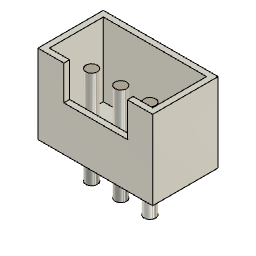
MLA30 v1.1 (Autodesk Fusion 360 archive; units mm, degrees)
design "JST-XH-3P"
Autodesk Fusion 360 part; units mm, degrees
note: some values were not read from the file. Set by a fixed rule: which face or edge a step refers to.
sketch "Esquisse1" plane through (0, 0, 0) normal (0, 0, 1) x (1, 0, 0) in component "JST-XH-3P"
  line L0 (6.25, 2.85) -> (-3.75, 2.85)
  line L1 (-3.75, 2.85) -> (-3.75, -2.85)
  line L2 (-3.75, -2.85) -> (6.25, -2.85)
  line L3 (6.25, -2.85) -> (6.25, 2.85)
  line L4 (6.25, 2.85) -> (-3.75, -2.85) construction
  line L5 (-3.75, 2.85) -> (6.25, -2.85) construction
  circle A0 centre (-1.27, -0.65) radius 0.5
  circle A1 centre (1.27, -0.65) radius 0.5
  circle A2 centre (3.81, -0.65) radius 0.5
  point P0 (1.25, 0)
  dimension "d6" = 10
  dimension "d7" = 5.7
  dimension "d8" = 1
  dimension "d11" = 5.08
  dimension "d12" = 0
  dimension "d13" = 2.48
  dimension "d20" = 2.2
  constraint horizontal L0
  constraint perpendicular L0 L1
  constraint parallel L0 L2
  constraint parallel L1 L3
  constraint coincident L4 P0
  constraint coincident L5 P0
  measures "d6" distance of L1.end L2.end
  measures "d7" distance of L0.end L1.end
  measures "d8" diameter of A0
  measures "d13" distance of L1 A0.centre
  measures "d20" distance of L2 A0.centre
extrude "Extrusion1" add sketch "Esquisse1" along normal blind 6.9 contours L0 L1 L2 L3 | A0 | A1 | A2 makes body 1 in component "JST-XH-3P"
shell "Coque1" thickness 0.5 removed faces 1 at (-0.4167, 0.95, 6.9) on bodies 1 in component "JST-XH-3P"
extrude "Extrusion2" add sketch "Esquisse1" against normal blind 3 separate body contours A0 | A1 | A2 makes body 2 at (-0.7706, -0.6749, -2) makes body 3 at (1.7694, -0.6749, -2) makes body 4 at (4.3094, -0.6749, -2) in component "JST-XH-3P"
sketch "Esquisse2" plane through (0, -2.85, 0) normal (0, -1, 0) x (1, 0, 0) in component "JST-XH-3P"
  line L0 (-3.75, 0) -> (6.25, 0)
  line L1 (6.25, 0) -> (6.25, 6.9)
  line L2 (6.25, 6.9) -> (-3.75, 6.9)
  line L3 (-3.75, 6.9) -> (-3.75, 0)
  line L4 (-1.4912, 6.9) -> (4.0488, 6.9)
  line L5 (4.0488, 6.9) -> (4.0488, 3.9)
  line L6 (4.0488, 3.9) -> (-1.4912, 3.9)
  line L7 (-1.4912, 3.9) -> (-1.4912, 6.9)
  dimension "d21" = 5.54
  dimension "d22" = 3
  constraint horizontal L4
  constraint vertical L5
  constraint horizontal L6
  constraint vertical L7
  constraint coincident L2 L4.start
  measures "d21" distance of L4.start L4.end
  measures "d22" distance of L4.start L6.end
extrude "Extrusion3" cut sketch "Esquisse2" against normal up to surface (0.5 mm away) contours L2 L4 L5 L6 L7 bodies 1 in component "JST-XH-3P"
extrude "Extrusion4" add sketch "Esquisse1" along normal blind 5.5 separate body contours A0 | A1 | A2 makes body 5 at (-0.7706, -0.6749, 3.6667) makes body 6 at (1.7694, -0.6749, 3.6667) makes body 7 at (4.3094, -0.6749, 3.6667) in component "JST-XH-3P"
component "JST-XH-3P" placed x (1, 0, 0) y (0, 1, 0) z (0, 0, 1) at (0, 0, 0)

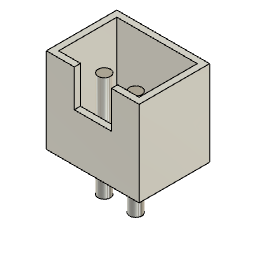
design "JST-XH-2P"
Autodesk Fusion 360 part; units mm, degrees
sketch "Esquisse1" plane through (0, 0, 0) normal (0, 0, 1) x (1, 0, 0) in component "JST-XH-2P"
  line L0 (3.75, 2.85) -> (-3.75, 2.85)
  line L1 (-3.75, 2.85) -> (-3.75, -2.85)
  line L2 (-3.75, -2.85) -> (3.75, -2.85)
  line L3 (3.75, -2.85) -> (3.75, 2.85)
  line L4 (3.75, 2.85) -> (-3.75, -2.85) construction
  line L5 (-3.75, 2.85) -> (3.75, -2.85) construction
  circle A0 centre (-1.27, -0.65) radius 0.5
  circle A1 centre (1.27, -0.65) radius 0.5
  dimension "d6" = 7.5
  dimension "d7" = 5.7
  dimension "d8" = 1
  dimension "d11" = 2.54
  dimension "d12" = 0
  dimension "d13" = 2.48
  dimension "d20" = 2.2
  constraint horizontal L0
  constraint perpendicular L0 L1
  constraint parallel L0 L2
  constraint parallel L1 L3
  constraint coincident L4 origin
  constraint coincident L5 origin
  measures "d6" distance of L1.end L2.end
  measures "d7" distance of L0.end L1.end
  measures "d8" diameter of A0
  measures "d13" distance of L1 A0.centre
  measures "d20" distance of L2 A0.centre
extrude "Extrusion1" add sketch "Esquisse1" along normal blind 6.9 contours L0 L1 L2 L3 | A0 | A1 makes body 1 in component "JST-XH-2P"
shell "Coque1" thickness 0.5 removed faces 1 at (-1.25, 0.95, 6.9) on bodies 1 in component "JST-XH-2P"
extrude "Extrusion2" add sketch "Esquisse1" against normal blind 3 separate body contours A0 | A1 makes body 2 at (-0.7706, -0.6749, -2) makes body 3 at (1.7694, -0.6749, -2) in component "JST-XH-2P"
sketch "Esquisse2" plane through (0, -2.85, 0) normal (0, -1, 0) x (1, 0, 0) in component "JST-XH-2P"
  line L0 (-3.75, 0) -> (3.75, 0)
  line L1 (3.75, 0) -> (3.75, 6.9)
  line L2 (3.75, 6.9) -> (-3.75, 6.9)
  line L3 (-3.75, 6.9) -> (-3.75, 0)
  line L4 (-1.4912, 6.9) -> (1.5088, 6.9)
  line L5 (1.5088, 6.9) -> (1.5088, 3.9)
  line L6 (1.5088, 3.9) -> (-1.4912, 3.9)
  line L7 (-1.4912, 3.9) -> (-1.4912, 6.9)
  dimension "d21" = 3
  dimension "d22" = 3
  constraint horizontal L4
  constraint vertical L5
  constraint horizontal L6
  constraint vertical L7
  constraint coincident L2 L4.start
  measures "d21" distance of L4.start L4.end
  measures "d22" distance of L4.start L6.end
extrude "Extrusion3" cut sketch "Esquisse2" against normal up to surface (0.5 mm away) contours L2 L4 L5 L6 L7 bodies 1 in component "JST-XH-2P"
extrude "Extrusion4" add sketch "Esquisse1" along normal blind 5.5 separate body contours A0 | A1 makes body 4 at (-0.7706, -0.6749, 3.6667) makes body 5 at (1.7694, -0.6749, 3.6667) in component "JST-XH-2P"
component "JST-XH-2P" placed x (1, 0, 0) y (0, 1, 0) z (0, 0, 1) at (0, 0, 0)

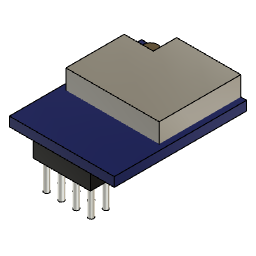
design "RA-02"
Autodesk Fusion 360 part; units mm, degrees
sketch "Esquisse1" plane through (0, 0, 0) normal (0, 0, 1) x (1, 0, 0) in component "LoRa RA-02"
  line L0 (0, 0) -> (18, 0)
  line L1 (18, 0) -> (18, -22.7)
  line L2 (18, -22.7) -> (0, -22.7)
  line L3 (0, -22.7) -> (0, 0)
  line L4 (1, 0) -> (17, 0)
  line L5 (17, 0) -> (17, -14)
  line L6 (17, -14) -> (1, -14)
  line L7 (1, -14) -> (1, 0)
  line L8 (13.9, -22.7) -> (4.1, -22.7)
  line L9 (4.1, -22.7) -> (4.1, -17.7)
  line L10 (4.1, -17.7) -> (13.9, -17.7)
  line L11 (13.9, -17.7) -> (13.9, -22.7)
  line L12 (1, 0) -> (6, 0)
  line L13 (6, 0) -> (6, -4)
  line L14 (6, -4) -> (1, -4)
  line L15 (1, -4) -> (1, 0)
  circle A0 centre (3.5142, -2) radius 1.25
  circle A1 centre (5.2, -21.5) radius 0.445
  circle A2 centre (7.74, -21.5) radius 0.445
  circle A3 centre (10.28, -21.5) radius 0.445
  circle A4 centre (12.82, -21.5) radius 0.445
  circle A5 centre (5.2, -18.96) radius 0.445
  circle A6 centre (7.74, -18.96) radius 0.445
  circle A7 centre (10.28, -18.96) radius 0.445
  circle A8 centre (12.82, -18.96) radius 0.445
  dimension "d1" = 18
  dimension "d2" = 22.7
  dimension "d3" = 16
  dimension "d4" = 14
  dimension "d5" = 9.8
  dimension "d6" = 5
  dimension "d7" = 5
  dimension "d8" = 4
  dimension "d9" = 2.5
  dimension "d18" = 0.89
  dimension "d21" = 7.62
  dimension "d22" = 2.54
  dimension "d23" = 1.2
  dimension "d24" = 1.1
  constraint horizontal L0
  constraint vertical L1
  constraint horizontal L2
  constraint vertical L3
  constraint coincident L0.start L3.end
  constraint horizontal L4
  constraint vertical L5
  constraint horizontal L6
  constraint vertical L7
  constraint coincident L0 L4.start
  constraint midpoint L0 L4
  constraint horizontal L8
  constraint vertical L9
  constraint horizontal L10
  constraint vertical L11
  constraint coincident L2 L8.start
  constraint midpoint L2 L8
  constraint horizontal L12
  constraint vertical L13
  constraint horizontal L14
  constraint vertical L15
  measures "d1" distance of L0.start L0.end
  measures "d2" distance of L0.start L2.end
  measures "d3" distance of L4.start L4.end
  measures "d4" distance of L4.start L6.end
  measures "d5" distance of L8.start L8.end
  measures "d6" distance of L8.start L10.end
  measures "d7" distance of L4.start L12.end
  measures "d8" distance of L4.start L14.end
  measures "d9" diameter of A0
  measures "d18" diameter of A1
  measures "d23" distance of L2 A1.centre
  measures "d24" distance of L9 A1.centre
extrude "Extrusion1" add sketch "Esquisse1" along normal blind 1.6 contours L0 L1 L2 L3 L5 L6 L7 L9 L10 L11 L15 | L0 L4 L7 L12 L13 L14 L15 | L0 L4 L5 L6 L7 L13 L14 | L2 L8 L9 L10 L11 | A0 | A1 | A2 | A3 | A4 | A5 | A6 | A7 | A8 makes body 1 in component "LoRa RA-02"
extrude "Extrusion2" add sketch "Esquisse1" against normal blind 2.6 separate body contours L2 L8 L9 L10 L11 | A1 | A2 | A3 | A4 | A5 | A6 | A7 | A8 makes body 2 in component "LoRa RA-02"
extrude "Extrusion3" add sketch "Esquisse1" along normal blind 4.9 separate body contours L0 L4 L5 L6 L7 L13 L14 makes body 3 in component "LoRa RA-02"
extrude "Extrusion4" add sketch "Esquisse1" along normal blind 3 separate body contours A0 makes body 4 in component "LoRa RA-02"
extrude "Extrusion5" add sketch "Esquisse1" against normal blind 5 from surface at -2.6 separate body contours A1 | A2 | A3 | A4 | A5 | A6 | A7 | A8 makes body 5 at (10.077, -19.356, -4.2667) makes body 6 at (8.1712, -21.6098, -5.9333) makes body 7 at (12.617, -21.896, -4.2667) makes body 8 at (8.1712, -19.0698, -5.9333) makes body 9 at (12.617, -19.356, -4.2667) makes body 10 at (5.6312, -21.6098, -5.9333) makes body 11 at (10.077, -21.896, -4.2667) makes body 12 at (5.6312, -19.0698, -5.9333) in component "LoRa RA-02"
component "LoRa RA-02" placed x (1, 0, 0) y (0, 1, 0) z (0, 0, 1) at (0, 0, 0)
named bodies: "PCB", "connecteur", "SX11278", "IPX"

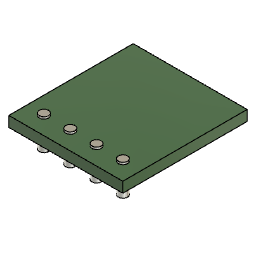
design "CRLD20MA"
Autodesk Fusion 360 part; units mm, degrees
sketch "Esquisse1" plane through (0, 0, 0) normal (0, 0, 1) x (1, 0, 0) in component "CRLD20MA"
  line L0 (5.5, -6) -> (-5.5, -6)
  line L1 (-5.5, -6) -> (-5.5, 6)
  line L2 (-5.5, 6) -> (5.5, 6)
  line L3 (5.5, 6) -> (5.5, -6)
  line L4 (5.5, -6) -> (-5.5, 6) construction
  line L5 (-5.5, -6) -> (5.5, 6) construction
  circle A0 centre (-3.81, -4.3) radius 0.4445
  circle A1 centre (-1.27, -4.3) radius 0.4445
  circle A2 centre (1.27, -4.3) radius 0.4445
  circle A3 centre (3.81, -4.3) radius 0.4445
  dimension "d1" = 11
  dimension "d2" = 12
  dimension "d3" = 0.889
  dimension "d6" = 7.62
  dimension "d7" = 0
  dimension "d8" = 1.7
  dimension "d9" = 1.69
  constraint horizontal L0
  constraint perpendicular L0 L1
  constraint parallel L0 L2
  constraint parallel L1 L3
  constraint coincident L4 origin
  constraint coincident L5 origin
  measures "d1" distance of L1.end L2.end
  measures "d2" distance of L0.end L1.end
  measures "d3" diameter of A0
  measures "d8" distance of L0 A0.centre
  measures "d9" distance of L1 A0.centre
extrude "Extrusion1" add sketch "Esquisse1" along normal blind 1 makes body 1 in component "CRLD20MA"
extrude "Extrusion2" add sketch "Esquisse1" against normal blind 3 from surface at 1.2 separate body contours A0 | A1 | A2 | A3 makes body 2 at (-0.8261, -4.3222, -0.8) makes body 3 at (1.7139, -4.3222, -0.8) makes body 4 at (-3.3661, -4.3222, -0.8) makes body 5 at (4.2539, -4.3222, -0.8) in component "CRLD20MA"
component "CRLD20MA" placed x (1, 0, 0) y (0, 1, 0) z (0, 0, 1) at (0, 0, 0)
